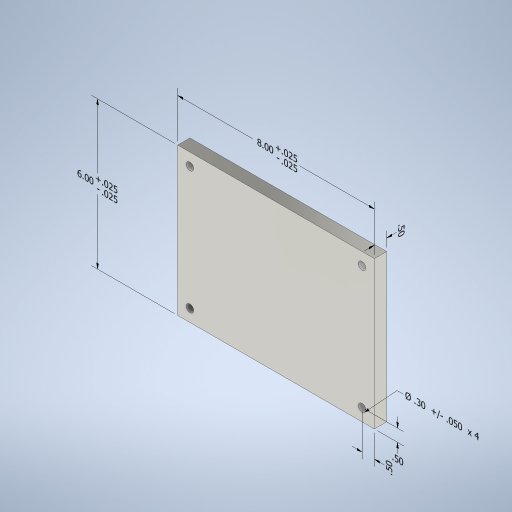
# Autodesk Inventor part: Base Plate
Saved by Autodesk Inventor 2023 (Build 270158000, 158)
## iProperties
Created: 2022-11-08
Part Number: Base Plate
Material: Generic
Document SubType Name: Modeling
Designer: 223076749
Density: 1 g/cm^3
Appearance: Default
Author: 223076749
Autodesk Inventor part; units mm, degrees
ref_plane "YZ Plane" through (0, 0, 0) normal (1, 0, 0) x (0, 1, 0)
ref_plane "XZ Plane" through (0, 0, 0) normal (0, 1, 0) x (-1, 0, 0)
ref_plane "XY Plane" through (0, 0, 0) normal (0, 0, 1) x (1, 0, 0)
sketch "Sketch1" plane through (0, 0, 0) normal (0, 0, 1) x (1, 0, 0)
  point P0 (0, 0)
sketch "Sketch2" plane through (0, 0, 0) normal (0, 0, 1) x (1, 0, 0)
  line L0 (0, 0) -> (203.2, 0)
  line L1 (203.2, 0) -> (203.2, 152.4)
  line L2 (203.2, 152.4) -> (0, 152.4)
  line L3 (0, 152.4) -> (0, 0)
  dimension "d1" = 203.2
  dimension "d2" = 152.4
  constraints: 8 end point, 2 parallel, 1 horizontal, 1 perpendicular
  measures "d1" distance of L2.end L1.end
  measures "d2" distance of L1.end L0.end
extrude "Extrusion1" add sketch "Sketch2" along normal blind 12.7
sketch "Sketch4" plane through (0, 0, 12.7) normal (0, 0, 1) x (1, 0, 0)
  line L0 (0, 152.4) -> (0, 0) projected
  line L1 (0, 0) -> (12.7, 0)
  line L2 (12.7, 0) -> (12.7, 12.7)
  line L3 (12.7, 12.7) -> (0, 12.7)
  line L4 (0, 12.7) -> (0, 0)
  line L5 (0, 0) -> (203.2, 0) projected
  line L6 (203.2, 0) -> (190.5, 0)
  line L7 (190.5, 0) -> (190.5, 12.7)
  line L8 (190.5, 12.7) -> (203.2, 12.7)
  line L9 (203.2, 12.7) -> (203.2, 0)
  line L10 (203.2, 0) -> (203.2, 152.4) projected
  line L11 (203.2, 152.4) -> (190.5, 152.4)
  line L12 (190.5, 152.4) -> (190.5, 139.7)
  line L13 (190.5, 139.7) -> (203.2, 139.7)
  line L14 (203.2, 139.7) -> (203.2, 152.4)
  line L15 (203.2, 152.4) -> (0, 152.4) projected
  line L16 (0, 152.4) -> (12.7, 152.4)
  line L17 (12.7, 152.4) -> (12.7, 139.7)
  line L18 (12.7, 139.7) -> (0, 139.7)
  line L19 (0, 139.7) -> (0, 152.4)
  dimension "d41" = 12.7
  dimension "d42" = 12.7
  dimension "d43" = 12.7
  dimension "d44" = 12.7
  dimension "d45" = 12.7
  dimension "d46" = 12.7
  dimension "d47" = 12.7
  dimension "d48" = 12.7
  constraints: 32 end point, 8 parallel, 4 horizontal, 4 perpendicular
  measures "d41" distance of L3.end L2.end
  measures "d42" distance of L7.end L8.end
  measures "d43" distance of L6.end L7.end
  measures "d44" distance of L13.end L12.end
  measures "d45" distance of L12.end L11.end
  measures "d46" distance of L17.end L18.end
  measures "d47" distance of L16.end L17.end
  measures "d48" distance between parallel lines of L5 L3
hole "Hole2" at (12.7, 139.7, 12.7) at (190.5, 139.7, 12.7) at (190.5, 12.7, 12.7) at (12.7, 12.7, 12.7) direction (0, 0, -1) diameter 7.62 end through all
body "Solid1"
